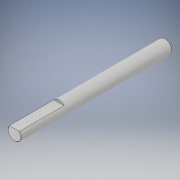
# Autodesk Inventor part: walek
Saved by Autodesk Inventor 2019 (Build 230136000, 136)
## iProperties
Created: 2020-05-17
Part Number: walek
Material: Generic
Document SubType Name: Modeling
Designer: estee
Density: 1 g/cm^3
Appearance: Default
Author: estee
Autodesk Inventor part; units mm, degrees
ref_plane "YZ Plane" through (0, 0, 0) normal (1, 0, 0) x (0, 1, 0)
ref_plane "XZ Plane" through (0, 0, 0) normal (0, 1, 0) x (-1, 0, 0)
ref_plane "XY Plane" through (0, 0, 0) normal (0, 0, 1) x (1, 0, 0)
sketch "Sketch1" plane through (0, 0, 0) normal (0, 0, 1) x (1, 0, 0)
  circle A0 centre (0, 0) radius 6
  dimension "d0" = 12
  constraints: 1 centre point, 1 coincident
  measures "d0" diameter of A0
extrude "Extrusion1" add sketch "Sketch1" along normal blind 135
chamfer "Chamfer1" distance 0.5 angle 45 2 edges at (-6, 0, 135) (-6, 0, 0)
sketch "Sketch2" plane through (0, 0, 135) normal (0, 0, 1) x (1, 0, 0)
  line L0 (-4.4614, 4) -> (4.4928, 4)
  point P0 (0, 0)
  dimension "d6" = 4
  constraints: 2 end point, 1 horizontal
  measures "d6" distance from line of L0 point (0, 0)
extrude "Extrusion2" cut sketch "Sketch2" against normal blind 40 fills toward (0.0157, 4.05) open curves L0
body "Solid1"
